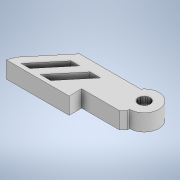
# Autodesk Inventor part: pinza  individuial sg996r con rosca
Saved by Autodesk Inventor 2021 (Build 250183000, 183)
## iProperties
Created: 2022-04-17
Part Number: pinza  individuial sg996r con rosca
Material: Genérico
Document SubType Name: Modeling
Designer: orgyn
Density: 1 g/cm^3
Appearance: Valor por defecto
Author: orgyn
Autodesk Inventor part; units mm, degrees
ref_plane "YZ Plane" through (0, 0, 0) normal (1, 0, 0) x (0, 1, 0)
ref_plane "XZ Plane" through (0, 0, 0) normal (0, 1, 0) x (-1, 0, 0)
ref_plane "XY Plane" through (0, 0, 0) normal (0, 0, 1) x (1, 0, 0)
sketch "Boceto1" plane through (0, 0, 0) normal (0, 1, 0) x (-1, 0, 0)
  line L0 (50, -16) -> (50, -16.5)
  line L1 (50, -16.5) -> (49.0807, -16.5)
  circle A0 centre (0, -33) radius 1.5
  circle A1 centre (0, -33) radius 3
  arc A2 (0, -26) -> (5.7446, -37) centre (0, -33) ccw
  line L2 (5.7446, -37) -> (35, -37)
  line L3 (35, -37) -> (50, -19)
  line L4 (0, -23) -> (20, -23)
  line L5 (20, -23) -> (20, -17)
  line L6 (20, -17) -> (50, -17)
  line L7 (50, -17) -> (50, -19)
  line L8 (0, -31.5) -> (0, -30)
  line L9 (0, -26) -> (0, -23)
  point P0 (0, -37)
  dimension "d9" = 0.5
  constraints: 20 end point, 3 coincident, 2 point on circle, 2 vertical alignment, 1 centre point, 1 perpendicular, 1 symmetric about line, 1 vertical, 4 other
  measures "d9" distance of L0.start L0.end
extrude "Extrusión1" add sketch "Boceto1" along normal blind 8 contours A1 | L9 L4 L5 L6 L7 L3 L2 A2
sketch "Boceto6" plane through (0, 0, 0) normal (0, -1, 0) x (1, 0, 0)
  line L0 (-50, -17) -> (-20, -17) projected
  line L1 (-50, -16) -> (-50, -14) projected
  line L2 (-50, -17) -> (-50, -16)
  line L3 (-50, -16.5) -> (-16.403, -16.5)
  line L4 (-20, -23) -> (-25, -23)
  line L5 (-5.7446, -37) -> (-35, -37) projected
  line L6 (-25, -23) -> (-25, -28)
  line L7 (-25, -37) -> (-25, -32)
  line L8 (-25, -32) -> (-5.7446, -32)
  line L9 (-5.7446, -32) -> (-5.7446, -27.061)
  line L10 (-25, -28) -> (-5.7446, -28)
  line L11 (-35, -37) -> (-30, -37)
  line L12 (-30, -37) -> (-30, -32)
  line L13 (-30, -32) -> (-25, -32)
  line L14 (-50, -19) -> (-50, -17) projected
  line L15 (-50, -19) -> (-45, -19)
  line L16 (-30, -37) -> (-45, -19)
  line L17 (-45, -19) -> (-40, -19)
  line L18 (-30, -32) -> (-40.8333, -19)
  line L19 (-40.8333, -19) -> (-25, -19)
  line L20 (-25, -19) -> (-25, -28)
  line L21 (-30, -32) -> (-34.1667, -32)
  line L22 (-40.8333, -19) -> (-35.8333, -19)
  line L23 (-35.8333, -19) -> (-25, -32)
  line L24 (-35.8333, -19) -> (-30.8333, -19)
  line L25 (-25, -32) -> (-20, -32)
  line L26 (-20, -32) -> (-30.8333, -19)
  line L27 (-30, 4) -> (-45, -14)
  line L28 (-45, -14) -> (-40, -14)
  line L29 (-30, -1) -> (-40.8333, -14)
  line L30 (-30, -1) -> (-34.1667, -1)
  line L31 (-35.8333, -14) -> (-25, -1)
  line L32 (-35.8333, -14) -> (-30.8333, -14)
  line L33 (-25, -1) -> (-20, -1)
  line L34 (-20, -1) -> (-30.8333, -14)
  point P0 (0, 0)
  dimension "d28" = 5
  dimension "d29" = 5
  dimension "d30" = 5
  dimension "d31" = 5
  dimension "d32" = 5
  dimension "d33" = 5
  dimension "d34" = 5
  dimension "d35" = 5
  dimension "d36" = 5
  constraints: 62 end point, 12 point on line, 10 symmetric about line, 5 perpendicular, 3 horizontal, 3 parallel, 2 vertical, 1 collinear, 1 midpoint
  measures "d28" distance of L4.start L4.end
  measures "d29" distance of L4.end L6.end
  measures "d30" distance of L7.start L7.end
  measures "d31" distance of L5.end L11.end
  measures "d32" distance of L14.start L15.end
  measures "d33" distance of L15.end L17.end
  measures "d34" distance of L18.end L22.end
  measures "d35" distance of L22.end L24.end
  measures "d36" distance of L7.end L25.end
extrude "Extrusión6" cut sketch "Boceto6" against normal blind 10 contours L23 L19 L26 L6 L10 L8 | L21 L16 L17 L18 | L10 L6 L26 | L30 L29 L28 L27 | L31 L33 L34 L32
chamfer "Chaflán1" distance 2 angle 45 2 edges at (-50, 4, -19) (0, 4, -23)
sketch "Boceto9" plane through (0, 8, 0) normal (0, 1, 0) x (1, 0, 0)
  circle A0 centre (0, 33) radius 1.5 projected
  circle A1 centre (0, 33) radius 2.6
  line L0 (0, 33) -> (0, 30.1)
  line L1 (0, 30.4) -> (0, 30.4753)
  line L2 (0, 30.4753) -> (0.263, 30.4753)
  line L3 (0.263, 30.4753) -> (-0.263, 30.4753)
  line L4 (-0.263, 30.4753) -> (-0.263, 29.9607)
  line L5 (0.263, 30.4753) -> (0.263, 30.0075)
  line L6 (0, 30.4) -> (0, 30.1)
  line L7 (0, 30.1) -> (0.263, 30.4133)
  line L8 (0, 30.1) -> (-0.263, 30.4133)
  line L9 (0.694, 30.1843) -> (0.8744, 30.5514)
  line L10 (0.694, 30.1843) -> (0.3637, 30.4256)
  line L11 (1.3477, 30.4322) -> (1.435, 30.8318)
  line L12 (1.3477, 30.4322) -> (0.9692, 30.5874)
  line L13 (1.9231, 30.8293) -> (1.9121, 31.2383)
  line L14 (1.9231, 30.8293) -> (1.5184, 30.8895)
  line L15 (2.3867, 31.3526) -> (2.2782, 31.7471)
  line L16 (2.3867, 31.3526) -> (1.9794, 31.3142)
  line L17 (2.7115, 31.9716) -> (2.5118, 32.3287)
  line L18 (2.7115, 31.9716) -> (2.3253, 31.8368)
  line L19 (2.8789, 32.6504) -> (2.5995, 32.9493)
  line L20 (2.8789, 32.6504) -> (2.5361, 32.4271)
  line L21 (2.8789, 33.3496) -> (2.5361, 33.5729)
  line L22 (2.8789, 33.3496) -> (2.5995, 33.0507)
  line L23 (2.7115, 34.0284) -> (2.3253, 34.1632)
  line L24 (2.7115, 34.0284) -> (2.5118, 33.6713)
  line L25 (2.3867, 34.6474) -> (1.9794, 34.6858)
  line L26 (2.3867, 34.6474) -> (2.2782, 34.2529)
  line L27 (1.9231, 35.1707) -> (1.5184, 35.1105)
  line L28 (1.9231, 35.1707) -> (1.9121, 34.7617)
  line L29 (1.3477, 35.5678) -> (0.9692, 35.4126)
  line L30 (1.3477, 35.5678) -> (1.435, 35.1682)
  line L31 (0.694, 35.8157) -> (0.3637, 35.5744)
  line L32 (0.694, 35.8157) -> (0.8744, 35.4486)
  line L33 (0, 35.9) -> (-0.263, 35.5867)
  line L34 (0, 35.9) -> (0.263, 35.5867)
  line L35 (-0.694, 35.8157) -> (-0.8744, 35.4486)
  line L36 (-0.694, 35.8157) -> (-0.3637, 35.5744)
  line L37 (-1.3477, 35.5678) -> (-1.435, 35.1682)
  line L38 (-1.3477, 35.5678) -> (-0.9692, 35.4126)
  line L39 (-1.9231, 35.1707) -> (-1.9121, 34.7617)
  line L40 (-1.9231, 35.1707) -> (-1.5184, 35.1105)
  line L41 (-2.3867, 34.6474) -> (-2.2782, 34.2529)
  line L42 (-2.3867, 34.6474) -> (-1.9794, 34.6858)
  line L43 (-2.7115, 34.0284) -> (-2.5118, 33.6713)
  line L44 (-2.7115, 34.0284) -> (-2.3253, 34.1632)
  line L45 (-2.8789, 33.3496) -> (-2.5995, 33.0507)
  line L46 (-2.8789, 33.3496) -> (-2.5361, 33.5729)
  line L47 (-2.8789, 32.6504) -> (-2.5361, 32.4271)
  line L48 (-2.8789, 32.6504) -> (-2.5995, 32.9493)
  line L49 (-2.7115, 31.9716) -> (-2.3253, 31.8368)
  line L50 (-2.7115, 31.9716) -> (-2.5118, 32.3287)
  line L51 (-2.3867, 31.3526) -> (-1.9794, 31.3142)
  line L52 (-2.3867, 31.3526) -> (-2.2782, 31.7471)
  line L53 (-1.9231, 30.8293) -> (-1.5184, 30.8895)
  line L54 (-1.9231, 30.8293) -> (-1.9121, 31.2383)
  line L55 (-1.3477, 30.4322) -> (-0.9692, 30.5874)
  line L56 (-1.3477, 30.4322) -> (-1.435, 30.8318)
  line L57 (-0.694, 30.1843) -> (-0.3637, 30.4256)
  line L58 (-0.694, 30.1843) -> (-0.8744, 30.5514)
  point P0 (0, 0)
  dimension "d47" = 5.2
  dimension "d48" = 2.9
  dimension "d49" = 0.263
  dimension "d50" = 0.526
  dimension "d51" = 0.3
  dimension "d54" = 360
  constraints: 118 end point, 5 point on line, 2 perpendicular, 2 vertical, 1 coincident, 1 collinear, 136 other
  measures "d48" distance of L0.start L0.end
  measures "d49" distance of L1.end L2.end
  measures "d50" distance of L2.end L3.end
  measures "d51" distance of L1.start L0.end
extrude "Extrusión9" cut sketch "Boceto9" against normal blind 2.9
